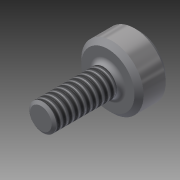
# Autodesk Inventor part: 13_2
Saved by Autodesk Inventor 2015 (Build 190159000, 159)
## iProperties
Created: 2015-03-31
Part Number: 13_2
Material: Generic
Document SubType Name: Modeling
Designer: WASHHSST
Density: 1 g/cm^3
Appearance: Default
Author: WASHHSST
Autodesk Inventor part; units mm, degrees
ref_plane "YZ Plane" through (0, 0, 0) normal (1, 0, 0) x (0, 1, 0)
ref_plane "XZ Plane" through (0, 0, 0) normal (0, 1, 0) x (-1, 0, 0)
ref_plane "XY Plane" through (0, 0, 0) normal (0, 0, 1) x (1, 0, 0)
sketch "Sketch2" plane through (0, 0, 0) normal (0, 0, 1) x (1, 0, 0)
  circle A0 centre (0, 0) radius 5.5499
  dimension "d3" = 11.0998
  constraints: 1 centre point, 1 coincident
  measures "d3" diameter of A0
extrude "Extrusion2" add sketch "Sketch2" along normal blind 5.5626
sketch "Sketch3" plane through (0, 0, 5.5626) normal (0, 0, 1) x (1, 0, 0)
  circle A0 centre (0, 0) radius 2.413
  dimension "d6" = 4.826
  constraints: 1 centre point, 1 coincident
  measures "d6" diameter of A0
extrude "Extrusion3" add sketch "Sketch3" along normal blind 11.9126
chamfer "Chamfer1" distance 0.4953 angle 35 1 edges at (-2.413, 0, 17.4752) measured on face at (0.8911, -0.3521, 17.4752)
thread "Thread1" size "10-24 UNC" class "2A" standard "ANSI Unified Screw Threads" full length
fillet "Fillet1" radius 0.8128 1 edges at (-2.413, 0, 5.5626)
chamfer "Chamfer2" distance 0.8128 angle 45 1 edges at (-5.5499, 0, 5.5626) measured on face at (4.7214, -0.4427, 5.5626)
chamfer "Chamfer3" distance 0.8128 angle 45 1 edges at (-5.5499, 0, 0) measured on face at (1.9719, 1.8895, 0)
body "Solid2"
